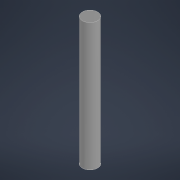
# Autodesk Inventor part: P005-Axe_piston
Saved by Autodesk Inventor 2021.3 (Build 253353000, 353)
## iProperties
Created: 2022-03-30
Part Number: P005-Axe_piston
Material: Aluminium
Document SubType Name: Modeling
Designer: Rémi & Elise
Density: 2.7 g/cm^3
Appearance: Aluminum - Dark
Mass: 0.477129 g
Surface Area: 2.49757 cm^2
Volume: 0.176715 cm^3
Author: Rémi & Elise
Title: Axe piston
Autodesk Inventor part; units mm, degrees
ref_plane "YZ Plane" through (0, 0, 0) normal (1, 0, 0) x (0, 1, 0)
ref_plane "XZ Plane" through (0, 0, 0) normal (0, 1, 0) x (-1, 0, 0)
ref_plane "XY Plane" through (0, 0, 0) normal (0, 0, 1) x (1, 0, 0)
sketch "Sketch2" plane through (0, 0, 0) normal (0, 0, 1) x (1, 0, 0)
  line L0 (-2.1, 0) -> (2.1, 0) construction
  line L1 (0, -2.1) -> (0, 2.1) construction
  circle A0 centre (0, 0) radius 1.5
  dimension "d0" = 3
  constraints: 1 centre point, 1 coincident
  measures "d0" diameter of A0
extrude "Extrusion1" add sketch "Sketch2" along normal blind 25
body "Solid1"
